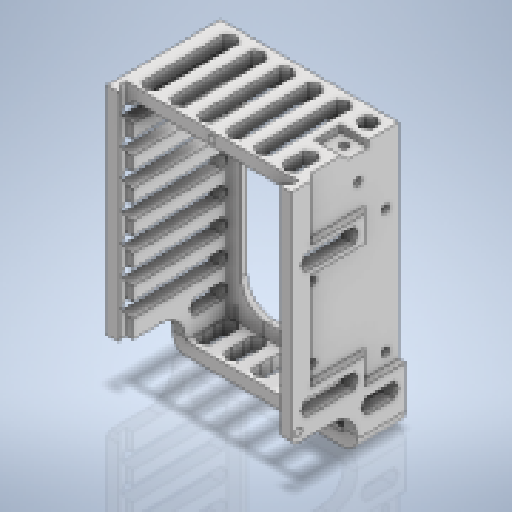
# Autodesk Inventor part: corpo
Saved by Autodesk Inventor 2024.3 (Build 283343000, 343)
## iProperties
Created: 2024-03-03
Part Number: corpo
Material: Genérico
Document SubType Name: Modeling
Designer: joaov
Density: 1 g/cm^3
Appearance: Padrão
Author: joaov
Autodesk Inventor part; units mm, degrees
note: some values were not read from the file. Chosen so that the rebuilt part matches the saved one: edges of "Chanfro6".
(part 1 of 2)
ref_plane "YZ Plane" through (0, 0, 0) normal (1, 0, 0) x (0, 1, 0)
ref_plane "XZ Plane" through (0, 0, 0) normal (0, 1, 0) x (-1, 0, 0)
ref_plane "XY Plane" through (0, 0, 0) normal (0, 0, 1) x (1, 0, 0)
sketch "Esboço1" plane through (0, 0, 0) normal (0, 0, 1) x (1, 0, 0)
  line L0 (0, 0) -> (59, 0)
  line L1 (59, 0) -> (59, 87)
  line L2 (59, 87) -> (0, 87)
  line L3 (0, 87) -> (0, 0)
  line L4 (59, 43.5) -> (63.8, 43.5)
  line L5 (29.5, 87) -> (29.5, 91.8)
  line L6 (-4.8, -4.8) -> (63.8, -4.8)
  line L7 (63.8, -4.8) -> (63.8, 91.8)
  line L8 (63.8, 91.8) -> (-4.8, 91.8)
  line L9 (-4.8, 91.8) -> (-4.8, -4.8)
  line L10 (-4.8, -4.8) -> (63.8, 91.8) construction
  line L11 (63.8, -4.8) -> (-4.8, 91.8) construction
  point P0 (29.5, 43.5)
  dimension "d0" = 59
  dimension "d1" = 87
  dimension "d2" = 4.8
  dimension "d3" = 4.8
  constraints: 24 end point, 4 midpoint, 4 perpendicular, 3 horizontal, 2 parallel, 1 vertical
  measures "d0" distance of L0.start L0.end
  measures "d1" distance of L0.end L1.end
  measures "d2" distance of L4.start L4.end
  measures "d3" distance of L5.start L5.end
extrude "paredes" add sketch "Esboço1" along normal blind 35 contours L0 L1 L4 L7 L6 L9 L8 L5 L2 L3 | L1 L2 L5 L8 L7 L4
sketch "Esboço2" plane through (0, 0, 0) normal (0, 0, -1) x (-1, 0, 0)
  line L0 (4.8, 91.8) -> (4.8, -4.8) projected
  line L1 (-63.8, 91.8) -> (4.8, 91.8)
  line L2 (4.8, 91.8) -> (4.8, -4.8)
  line L3 (4.8, -4.8) -> (-63.8, -4.8)
  line L4 (-63.8, -4.8) -> (-63.8, 91.8)
  point P0 (0, 0)
  constraints: 8 end point, 2 parallel, 1 horizontal, 1 perpendicular
extrude "base" add sketch "Esboço2" along normal blind 2.4
sketch "Esboço3" plane through (-4.8, -4.8, 35) normal (0, -1, 0) x (1, 0, 0)
  line L0 (0, -37.4) -> (0, 0) projected
  line L1 (0, 0) -> (2.4, 0)
  line L2 (68.6, 0) -> (0, 0) projected
  line L3 (0, 0) -> (0, 4.8)
  line L4 (0, 4.8) -> (4.3, 4.8)
  line L5 (2.4, 2.4) -> (4.3, 4.3)
  line L6 (2.4, 0) -> (2.4, 2.4)
  line L7 (4.3, 4.8) -> (4.3, 4.3)
  line L8 (34.3, 0) -> (34.3, 4.8)
  line L9 (68.6, 0) -> (66.2, 0)
  line L10 (68.6, 0) -> (68.6, 4.8)
  line L11 (68.6, 4.8) -> (64.3, 4.8)
  line L12 (66.2, 2.4) -> (64.3, 4.3)
  line L13 (66.2, 0) -> (66.2, 2.4)
  line L14 (64.3, 4.8) -> (64.3, 4.3)
  point P0 (4.8, -35)
  dimension "d27" = 0.5
  constraints: 26 end point, 5 symmetric about line, 2 vertical, 1 midpoint, 1 perpendicular, 1 point on line
  measures "d27" distance of L12.end L11.end
extrude "Extrusão3" add sketch "Esboço3" against normal blind 96.6
sketch "Esboço4" plane through (0, 0, 35) normal (0, 0, 1) x (1, 0, 0)
  line L0 (59, 87) -> (0, 87)
  line L1 (29.5, 87) -> (29.5, 91.8)
  line L2 (63.8, 91.8) -> (-4.8, 91.8)
  line L3 (29.5, 89.4) -> (51, 89.4)
  line L4 (29.5, 87) -> (29.5, 91.8)
  line L5 (29.5, 89.4) -> (8, 89.4)
  line L6 (29.5, 89.4) -> (51, 89.4)
  circle A0 centre (51, 89.4) radius 1.45
  circle A1 centre (8, 89.4) radius 1.45
  line L7 (59.5, -4.8) -> (59.5, 91.8) projected
  line L8 (-0.5, -4.8) -> (-0.5, 91.8) projected
  circle A2 centre (29.5, 89.4) radius 1.45
  point P0 (0, 0)
  point P1 (59, 0)
  point P2 (63.8, -4.8)
  point P3 (-4.8, -4.8)
  dimension "d161" = 8.5
  dimension "d162" = 8.5
  dimension "d255" = 2.9
  dimension "d265" = 2.9
  dimension "d266" = 2.9
  constraints: 14 end point, 3 centre point, 3 coincident
  measures "d161" distance from line of L3.end L7
  measures "d162" distance from line of L5.end L8
  measures "d255" diameter of A2
  measures "d265" diameter of A1
  measures "d266" diameter of A0
extrude "Extrusão4" cut sketch "Esboço4" against normal blind 10 contours A2 L5 L1 | L1 L3 A2 | L5 A2 L1 | L1 A2 L3
sketch "Esboço5" plane through (-4.8, -4.8, -2.4) normal (0, -1, 0) x (1, 0, 0)
  line L0 (0, 0) -> (68.6, 0) projected
  line L1 (20.3, 17.9) -> (10.3, 17.9)
  line L2 (20.3, 17.9) -> (30.3, 17.9)
  line L3 (30.3, 17.9) -> (20.3, 27.9)
  line L4 (20.3, 27.9) -> (10.3, 17.9)
  line L5 (66.2, 37.4) -> (2.4, 37.4) projected
  line L6 (2.4, 37.4) -> (2.4, 17.9)
  line L7 (4.8, 2.4) -> (4.8, 37.4) projected
  line L8 (2.4, 17.9) -> (66.2, 17.9)
  line L9 (66.2, 17.9) -> (66.2, 37.4)
  line L10 (66.2, 37.4) -> (2.4, 37.4)
  line L11 (0, 42.2) -> (4.3, 42.2) projected
  line L12 (68.6, 0) -> (68.6, 42.2) projected
  line L13 (0, 42.2) -> (68.6, 42.2)
  line L14 (68.6, 42.2) -> (68.6, 17.9)
  line L15 (68.6, 17.9) -> (0, 17.9)
  line L16 (0, 17.9) -> (0, 42.2)
  point P0 (2.4, 17.9)
  dimension "d36" = 10
  dimension "d37" = 10
  dimension "d38" = 45
  constraints: 24 end point, 5 perpendicular, 3 horizontal, 3 parallel, 1 point on line
  measures "d36" distance of L1.start L1.end
  measures "d37" distance of L1.start L2.end
  measures "d38" angle of L3 L2
extrude "Extrusão5" cut sketch "Esboço5" against normal blind 14.8
sketch "Esboço10" plane through (63.8, -4.8, -2.4) normal (1, 0, 0) x (0, 0, -1)
  line L0 (-7.5, 75.981) -> (0, 75.981)
  line L1 (-7.5, 20.619) -> (0, 20.619)
  line L2 (-7.5, 75.981) -> (-15.2, 75.981)
  line L3 (-15.2, 75.981) -> (-15.2, 66.3)
  line L4 (-15.2, 30.3) -> (-15.2, 20.619)
  line L5 (-15.2, 20.619) -> (-7.5, 20.619)
  line L6 (0, 75.981) -> (0, 20.619)
  line L7 (-18.58, 30.3) -> (-15.2, 30.3)
  line L8 (-18.58, 66.3) -> (-15.2, 66.3)
  line L9 (-35.3, 30.3) -> (-35.3, 66.3)
  line L10 (-18.58, 66.3) -> (-35.3, 66.3)
  line L11 (-18.58, 30.3) -> (-35.3, 30.3)
  line L12 (0, 0) -> (0, 96.6) projected
  line L13 (0, 96.6) -> (0, 0)
  point P0 (-2.4, 4.8)
  point P1 (-35.0419, -145.2014)
  constraints: 26 end point, 6 perpendicular, 1 collinear
extrude "Extrusão9" cut sketch "Esboço10" against normal blind 2.5
sketch "Esboço11" plane through (61.3, -4.8, -2.4) normal (1, 0, 0) x (0, 0, -1)
  line L0 (-15.2, 66.3) -> (-15.2, 75.981)
  line L1 (-15.2, 71.1405) -> (-15, 71.1405)
  line L2 (-15.2, 71.1405) -> (-15.2, 70.9405) construction
  line L3 (-15.2, 75.981) -> (0, 75.981)
  line L4 (-7.6, 75.981) -> (-7.6, 75.781)
  line L5 (-7.6, 75.981) -> (-7.6, 75.781) construction
  line L6 (0, 75.981) -> (0, 20.619)
  line L7 (0, 75.781) -> (-10, 75.781)
  line L8 (-5, 75.781) -> (-5, 72.781)
  line L9 (-5, 72.781) -> (-5, 71.281)
  line L10 (0, 48.3) -> (-3.0797, 48.3)
  line L11 (-15.2, 75.981) -> (0, 75.981)
  line L12 (-35.3, 66.3) -> (-15.2, 66.3)
  line L13 (-35.3, 30.3) -> (-35.3, 66.3)
  line L14 (-35.3, 66.3) -> (-35.3, 30.3)
  line L15 (-35.3, 48.3) -> (-32.1, 48.3)
  line L16 (-32.1, 66.3) -> (-32.1, 63.1)
  line L17 (-32.1, 63.1) -> (-32.1, 61.6)
  line L18 (0, 48.3) -> (-35.3, 48.3)
  line L19 (-17.65, 48.3) -> (-17.65, 54.676)
  line L20 (-35.3, 30.3) -> (-35.3, 66.3) projected
  line L21 (-35.3, 48.3) -> (-37.5242, 48.3)
  line L22 (-5, 25.319) -> (-15.2, 25.319)
  line L23 (-15.2, 20.619) -> (-15.2, 30.3) projected
  circle A0 centre (-5, 25.319) radius 1.45
  circle A1 centre (-32.1, 35) radius 1.45
  circle A2 centre (-32.1, 61.6) radius 1.45
  circle A3 centre (-5, 71.281) radius 1.45
  point P0 (-2.4, 4.8)
  point P1 (33.1289, 48.912)
  dimension "d58" = 90
  dimension "d59" = 0.2
  dimension "d61" = 3
  dimension "d62" = 1.5
  dimension "d64" = 3.2
  dimension "d65" = 3.2
  dimension "d66" = 1.5
  dimension "d260" = 2.9
  dimension "d261" = 2.9
  dimension "d262" = 2.9
  dimension "d263" = 2.9
  constraints: 44 end point, 8 midpoint, 4 centre point, 4 point on line, 2 equal length, 2 horizontal, 1 coincident, 1 perpendicular
  measures "d58" angle of L2 L1
  measures "d59" distance of L1.start L1.end
  measures "d61" distance of L8.start L8.end
  measures "d62" distance of L8.end L9.end
  measures "d64" distance of L15.start L15.end
  measures "d65" distance of L16.start L16.end
  measures "d66" distance of L16.end L17.end
  measures "d260" diameter of A0
  measures "d261" diameter of A1
  measures "d262" diameter of A2
  measures "d263" diameter of A3
extrude "Extrusão10" cut sketch "Esboço11" against normal blind 8.25 contours A0 | A1 | A2 | A3
chamfer "Chanfro1" distance 2.5 angle 45 1 edges at (61.3, 43.5, 32.9)
chamfer "Chanfro2" distance 2.5 angle 45 2 edges at (61.3, 20.6595, 12.8) (61.3, 66.3405, 12.8)
sketch "Esboço14" plane through (63.8, 91.8, 39.8) normal (1, 0, 0) x (0, 0, -1)
  line L0 (0, 0) -> (42.2, 0) projected
  line L1 (10.6384, 0) -> (38.6384, 0) construction
  line L2 (2.4, -81.8) -> (2.4, 0) projected
  line L3 (2.4, 0) -> (2.4, -30.2771)
  line L4 (2.4, -30.2771) -> (4.8, -30.2771)
  line L5 (4.8, -4.8) -> (4.8, -81.8) projected
  line L6 (4.8, -30.2771) -> (4.8, 0)
  line L7 (6.9, -66.3) -> (6.9, -30.3) projected
  line L8 (6.9, -20.619) -> (6.9, 0)
  line L9 (27, -30.3) -> (27, -20.619) projected
  line L10 (27, -20.619) -> (6.9, -20.619)
  line L11 (42.2, 0) -> (42.2, -20.619) projected
  line L12 (42.2, -20.619) -> (27, -20.619)
  line L13 (42.2, -20.619) -> (42.2, 0)
  line L14 (0, 0) -> (6.9, 0)
  line L15 (42.2, 0) -> (0, 0) projected
  line L16 (6.9, 0) -> (42.2, 0)
  point P0 (39.8, -91.8)
  dimension "d101" = 35.3
  dimension "d102" = 20.619
  constraints: 20 end point, 4 perpendicular, 4 point on line, 3 horizontal, 2 collinear, 1 vertical
  measures "d101" distance of L0.end L8.end
  measures "d102" distance of L0.end L11.end
extrude "Extrusão11" cut sketch "Esboço14" against normal blind 2.5 contours L0 L11 L12 L10 L8
chamfer "Chanfro3" distance 2.5 angle 45 1 edges at (61.3, 81.4905, 32.9)
sketch "Esboço17" plane through (-2.4, 91.8, 35) normal (0, 1, 0) x (1, 0, 0)
  line L0 (53.7, 21) -> (53.7, 16)
  line L1 (53.7, 16) -> (63.7, 16)
  line L2 (63.7, 16) -> (63.7, 26)
  line L3 (63.7, 26) -> (53.7, 26)
  line L4 (53.7, 26) -> (53.7, 21)
  point P0 (63.7, 4.6)
  constraints: 10 end point, 1 horizontal, 1 perpendicular, 1 vertical
extrude "Extrusão14" cut sketch "Esboço17" against normal blind 2.5
chamfer "Chanfro6" distance 2.5 angle 45 1 edges at (56.3, 89.3, 19)
sketch "Esboço18" plane through (-2.4, 89.3, 35) normal (0, 1, 0) x (1, 0, 0)
  line L0 (2.4, 0) -> (61.4, 0) projected
  line L1 (-2.4, 37.4) -> (63.7, 37.4) projected
  circle A0 centre (58.7, 22.25) radius 1.45
  point P0 (10.1, 26)
  point P1 (0.1, 18.5)
  dimension "d264" = 2.9
  constraints: 1 centre point
  measures "d264" diameter of A0
extrude "Extrusão15" cut sketch "Esboço18" against normal blind 2.5
fillet "Arredondamento2" radius 9 2 edges at (-2.4, 10, 15.5) (61.4, 10, 15.5)
fillet "Arredondamento3" radius 5 2 edges at (-4.8, -4.8, 6.55) (63.8, -4.8, 6.55)
sketch "Esboço24" plane through (-4.8, 91.8, -2.4) normal (-1, 0, 0) x (0, 0, 1)
  line L0 (28.975, -77) -> (35, -77)
  line L1 (-2.4, -30.2362) -> (2.4, -30.2362) construction
  line L2 (2.4, -9.5605) -> (4.03, -6.7373)
  line L3 (4.03, -6.7373) -> (7.29, -6.7373)
  line L4 (7.29, -6.7373) -> (8.92, -9.5605)
  line L5 (8.92, -9.5605) -> (7.29, -12.3838)
  line L6 (7.29, -12.3838) -> (4.03, -12.3838)
  line L7 (4.03, -12.3838) -> (2.4, -9.5605)
  line L8 (2.4, -20.007) -> (4.03, -17.1838)
  line L9 (4.03, -17.1838) -> (7.29, -17.1838)
  line L10 (7.29, -17.1838) -> (8.92, -20.007)
  line L11 (8.92, -20.007) -> (7.29, -22.8303)
  line L12 (7.29, -22.8303) -> (4.03, -22.8303)
  line L13 (4.03, -22.8303) -> (2.4, -20.007)
  line L14 (2.4, -30.4535) -> (4.03, -27.6303)
  line L15 (4.03, -27.6303) -> (7.29, -27.6303)
  line L16 (7.29, -27.6303) -> (8.92, -30.4535)
  line L17 (8.92, -30.4535) -> (7.29, -33.2768)
  line L18 (7.29, -33.2768) -> (4.03, -33.2768)
  line L19 (4.03, -33.2768) -> (2.4, -30.4535)
  line L20 (7.29, -43.7232) -> (4.03, -43.7232)
  line L21 (8.92, -40.9) -> (7.29, -43.7232)
  line L22 (4.03, -43.7232) -> (2.4, -40.9)
  line L23 (2.4, -40.9) -> (4.03, -38.0768)
  line L24 (4.03, -38.0768) -> (7.29, -38.0768)
  line L25 (7.29, -38.0768) -> (8.92, -40.9)
  line L26 (2.4, -51.3465) -> (4.03, -48.5232)
  line L27 (4.03, -48.5232) -> (7.29, -48.5232)
  line L28 (7.29, -48.5232) -> (8.92, -51.3465)
  line L29 (8.92, -51.3465) -> (7.29, -54.1697)
  line L30 (7.29, -54.1697) -> (4.03, -54.1697)
  line L31 (4.03, -54.1697) -> (2.4, -51.3465)
  line L32 (7.29, -64.6162) -> (4.03, -64.6162)
  line L33 (8.92, -61.793) -> (7.29, -64.6162)
  line L34 (4.03, -64.6162) -> (2.4, -61.793)
  line L35 (2.4, -61.793) -> (4.03, -58.9697)
  line L36 (4.03, -58.9697) -> (7.29, -58.9697)
  line L37 (7.29, -58.9697) -> (8.92, -61.793)
  line L38 (4.03, -69.4162) -> (7.29, -69.4162)
  line L39 (2.4, -72.2395) -> (4.03, -69.4162)
  line L40 (4.03, -75.0627) -> (2.4, -72.2395)
  line L41 (7.29, -69.4162) -> (8.92, -72.2395)
  line L42 (7.29, -75.0627) -> (4.03, -75.0627)
  line L43 (8.92, -72.2395) -> (7.29, -75.0627)
  line L44 (4.03, -79.8627) -> (7.29, -79.8627)
  line L45 (4.03, -85.5092) -> (2.4, -82.6859)
  line L46 (7.29, -85.5092) -> (4.03, -85.5092)
  line L47 (2.4, -82.6859) -> (4.03, -79.8627)
  line L48 (7.29, -79.8627) -> (8.92, -82.6859)
  line L49 (8.92, -82.6859) -> (7.29, -85.5092)
  line L50 (8.92, -9.5605) -> (9.92, -9.5605)
  line L51 (9.92, -9.5605) -> (11.55, -6.7373)
  line L52 (11.55, -6.7373) -> (14.81, -6.7373)
  line L53 (14.81, -6.7373) -> (16.44, -9.5605)
  line L54 (16.44, -9.5605) -> (14.81, -12.3838)
  line L55 (14.81, -12.3838) -> (11.55, -12.3838)
  line L56 (11.55, -12.3838) -> (9.92, -9.5605)
  line L57 (14.81, -22.8303) -> (11.55, -22.8303)
  line L58 (16.44, -20.007) -> (14.81, -22.8303)
  line L59 (11.55, -22.8303) -> (9.92, -20.007)
  line L60 (9.92, -20.007) -> (11.55, -17.1838)
  line L61 (11.55, -17.1838) -> (14.81, -17.1838)
  line L62 (14.81, -17.1838) -> (16.44, -20.007)
  line L63 (9.92, -30.4535) -> (11.55, -27.6303)
  line L64 (11.55, -27.6303) -> (14.81, -27.6303)
  line L65 (14.81, -27.6303) -> (16.44, -30.4535)
  line L66 (16.44, -30.4535) -> (14.81, -33.2768)
  line L67 (14.81, -33.2768) -> (11.55, -33.2768)
  line L68 (11.55, -33.2768) -> (9.92, -30.4535)
  line L69 (14.81, -43.7232) -> (11.55, -43.7232)
  line L70 (16.44, -40.9) -> (14.81, -43.7232)
  line L71 (11.55, -43.7232) -> (9.92, -40.9)
  line L72 (14.81, -38.0768) -> (16.44, -40.9)
  line L73 (11.55, -38.0768) -> (14.81, -38.0768)
  line L74 (9.92, -40.9) -> (11.55, -38.0768)
  line L75 (9.92, -51.3465) -> (11.55, -48.5232)
  line L76 (11.55, -48.5232) -> (14.81, -48.5232)
  line L77 (14.81, -48.5232) -> (16.44, -51.3465)
  line L78 (16.44, -51.3465) -> (14.81, -54.1697)
  line L79 (14.81, -54.1697) -> (11.55, -54.1697)
  line L80 (11.55, -54.1697) -> (9.92, -51.3465)
  line L81 (14.81, -64.6162) -> (11.55, -64.6162)
  line L82 (16.44, -61.793) -> (14.81, -64.6162)
  line L83 (11.55, -64.6162) -> (9.92, -61.793)
  line L84 (14.81, -58.9697) -> (16.44, -61.793)
  line L85 (11.55, -58.9697) -> (14.81, -58.9697)
  line L86 (9.92, -61.793) -> (11.55, -58.9697)
  line L87 (11.55, -69.4162) -> (14.81, -69.4162)
  line L88 (11.55, -75.0627) -> (9.92, -72.2395)
  line L89 (14.81, -75.0627) -> (11.55, -75.0627)
  line L90 (9.92, -72.2395) -> (11.55, -69.4162)
  line L91 (14.81, -69.4162) -> (16.44, -72.2395)
  line L92 (16.44, -72.2395) -> (14.81, -75.0627)
  line L93 (11.55, -79.8627) -> (14.81, -79.8627)
  line L94 (14.81, -79.8627) -> (16.44, -82.6859)
  line L95 (9.92, -82.6859) -> (11.55, -79.8627)
  line L96 (16.44, -82.6859) -> (14.81, -85.5092)
  line L97 (14.81, -85.5092) -> (11.55, -85.5092)
  line L98 (11.55, -85.5092) -> (9.92, -82.6859)
  line L99 (16.44, -9.5605) -> (17.44, -9.5605)
  line L100 (17.44, -9.5605) -> (19.07, -6.7373)
  line L101 (19.07, -6.7373) -> (22.33, -6.7373)
  line L102 (22.33, -6.7373) -> (23.96, -9.5605)
  line L103 (23.96, -9.5605) -> (22.33, -12.3838)
  line L104 (22.33, -12.3838) -> (19.07, -12.3838)
  line L105 (19.07, -12.3838) -> (17.44, -9.5605)
  line L106 (22.33, -22.8303) -> (19.07, -22.8303)
  line L107 (23.96, -20.007) -> (22.33, -22.8303)
  line L108 (19.07, -22.8303) -> (17.44, -20.007)
  line L109 (17.44, -20.007) -> (19.07, -17.1838)
  line L110 (19.07, -17.1838) -> (22.33, -17.1838)
  line L111 (22.33, -17.1838) -> (23.96, -20.007)
  line L112 (17.44, -30.4535) -> (19.07, -27.6303)
  line L113 (19.07, -27.6303) -> (22.33, -27.6303)
  line L114 (22.33, -27.6303) -> (23.96, -30.4535)
  line L115 (23.96, -30.4535) -> (22.33, -33.2768)
  line L116 (22.33, -33.2768) -> (19.07, -33.2768)
  line L117 (19.07, -33.2768) -> (17.44, -30.4535)
  line L118 (22.33, -43.7232) -> (19.07, -43.7232)
  line L119 (23.96, -40.9) -> (22.33, -43.7232)
  line L120 (19.07, -43.7232) -> (17.44, -40.9)
  line L121 (22.33, -38.0768) -> (23.96, -40.9)
  line L122 (19.07, -38.0768) -> (22.33, -38.0768)
  line L123 (17.44, -40.9) -> (19.07, -38.0768)
  line L124 (17.44, -51.3465) -> (19.07, -48.5232)
  line L125 (19.07, -48.5232) -> (22.33, -48.5232)
  line L126 (22.33, -48.5232) -> (23.96, -51.3465)
  line L127 (23.96, -51.3465) -> (22.33, -54.1697)
  line L128 (22.33, -54.1697) -> (19.07, -54.1697)
  line L129 (19.07, -54.1697) -> (17.44, -51.3465)
  line L130 (22.33, -64.6162) -> (19.07, -64.6162)
  line L131 (23.96, -61.793) -> (22.33, -64.6162)
  line L132 (19.07, -64.6162) -> (17.44, -61.793)
  line L133 (22.33, -58.9697) -> (23.96, -61.793)
  line L134 (19.07, -58.9697) -> (22.33, -58.9697)
  line L135 (17.44, -61.793) -> (19.07, -58.9697)
  line L136 (19.07, -69.4162) -> (22.33, -69.4162)
  line L137 (19.07, -75.0627) -> (17.44, -72.2395)
  line L138 (22.33, -75.0627) -> (19.07, -75.0627)
  line L139 (17.44, -72.2395) -> (19.07, -69.4162)
  line L140 (22.33, -69.4162) -> (23.96, -72.2395)
  line L141 (23.96, -72.2395) -> (22.33, -75.0627)
  line L142 (23.96, -9.5605) -> (24.96, -9.5605)
  line L143 (24.96, -9.5605) -> (26.59, -6.7373)
  line L144 (26.59, -6.7373) -> (29.85, -6.7373)
  line L145 (29.85, -6.7373) -> (31.48, -9.5605)
  line L146 (31.48, -9.5605) -> (29.85, -12.3838)
  line L147 (29.85, -12.3838) -> (26.59, -12.3838)
  line L148 (26.59, -12.3838) -> (24.96, -9.5605)
  line L149 (29.85, -22.8303) -> (26.59, -22.8303)
  line L150 (31.48, -20.007) -> (29.85, -22.8303)
  line L151 (26.59, -22.8303) -> (24.96, -20.007)
  line L152 (24.96, -20.007) -> (26.59, -17.1838)
  line L153 (26.59, -17.1838) -> (29.85, -17.1838)
  line L154 (29.85, -17.1838) -> (31.48, -20.007)
  line L155 (24.96, -30.4535) -> (26.59, -27.6303)
  line L156 (26.59, -27.6303) -> (29.85, -27.6303)
  line L157 (29.85, -27.6303) -> (31.48, -30.4535)
  line L158 (31.48, -30.4535) -> (29.85, -33.2768)
  line L159 (29.85, -33.2768) -> (26.59, -33.2768)
  line L160 (26.59, -33.2768) -> (24.96, -30.4535)
  line L161 (29.85, -43.7232) -> (26.59, -43.7232)
  line L162 (31.48, -40.9) -> (29.85, -43.7232)
  line L163 (26.59, -43.7232) -> (24.96, -40.9)
  line L164 (29.85, -38.0768) -> (31.48, -40.9)
  line L165 (26.59, -38.0768) -> (29.85, -38.0768)
  line L166 (24.96, -40.9) -> (26.59, -38.0768)
  line L167 (24.96, -51.3465) -> (26.59, -48.5232)
  line L168 (26.59, -48.5232) -> (29.85, -48.5232)
  line L169 (29.85, -48.5232) -> (31.48, -51.3465)
  line L170 (31.48, -51.3465) -> (29.85, -54.1697)
  line L171 (29.85, -54.1697) -> (26.59, -54.1697)
  line L172 (26.59, -54.1697) -> (24.96, -51.3465)
  line L173 (29.85, -64.6162) -> (26.59, -64.6162)
  line L174 (31.48, -61.793) -> (29.85, -64.6162)
  line L175 (26.59, -64.6162) -> (24.96, -61.793)
  line L176 (29.85, -58.9697) -> (31.48, -61.793)
  line L177 (26.59, -58.9697) -> (29.85, -58.9697)
  line L178 (24.96, -61.793) -> (26.59, -58.9697)
  line L179 (26.59, -69.4162) -> (29.85, -69.4162)
  line L180 (26.59, -75.0627) -> (24.96, -72.2395)
  line L181 (29.85, -75.0627) -> (26.59, -75.0627)
  line L182 (24.96, -72.2395) -> (26.59, -69.4162)
  line L183 (29.85, -69.4162) -> (31.48, -72.2395)
  line L184 (31.48, -72.2395) -> (29.85, -75.0627)
  line L185 (31.48, -9.5605) -> (32.48, -9.5605)
  line L186 (2.4, -9.5605) -> (0, -9.5605)
  line L187 (37.37, -33.2768) -> (34.11, -33.2768)
  line L188 (34.11, -33.2768) -> (32.48, -30.4535)
  line L189 (34.11, -27.6303) -> (37.37, -27.6303)
  line L190 (32.48, -30.4535) -> (34.11, -27.6303)
  line L191 (34.11, -38.0768) -> (37.37, -38.0768)
  line L192 (37.37, -38.0768) -> (39, -40.9)
  line L193 (32.48, -40.9) -> (34.11, -38.0768)
  line L194 (39, -40.9) -> (37.37, -43.7232)
  line L195 (37.37, -43.7232) -> (34.11, -43.7232)
  line L196 (34.11, -43.7232) -> (32.48, -40.9)
  line L197 (37.37, -27.6303) -> (39, -30.4535)
  line L198 (39, -30.4535) -> (37.37, -33.2768)
  line L199 (34.11, -48.5232) -> (37.37, -48.5232)
  line L200 (32.48, -51.3465) -> (34.11, -48.5232)
  line L201 (39, -51.3465) -> (37.37, -54.1697)
  line L202 (37.37, -54.1697) -> (34.11, -54.1697)
  line L203 (34.11, -54.1697) -> (32.48, -51.3465)
  line L204 (34.11, -58.9697) -> (37.37, -58.9697)
  line L205 (32.48, -61.793) -> (34.11, -58.9697)
  line L206 (37.37, -58.9697) -> (39, -61.793)
  line L207 (34.11, -64.6162) -> (32.48, -61.793)
  line L208 (37.37, -64.6162) -> (34.11, -64.6162)
  line L209 (39, -61.793) -> (37.37, -64.6162)
  line L210 (37.37, -48.5232) -> (39, -51.3465)
  line L211 (34.11, -69.4162) -> (37.37, -69.4162)
  line L212 (32.48, -72.2395) -> (34.11, -69.4162)
  line L213 (37.37, -69.4162) -> (39, -72.2395)
  line L214 (37.37, -75.0627) -> (34.11, -75.0627)
  line L215 (39, -72.2395) -> (37.37, -75.0627)
  line L216 (34.11, -75.0627) -> (32.48, -72.2395)
  line L217 (32.48, -9.5605) -> (34.11, -6.7373)
  line L218 (34.11, -6.7373) -> (37.37, -6.7373)
  line L219 (37.37, -6.7373) -> (39, -9.5605)
  line L220 (39, -9.5605) -> (37.37, -12.3838)
  line L221 (37.37, -12.3838) -> (34.11, -12.3838)
  line L222 (34.11, -12.3838) -> (32.48, -9.5605)
  line L223 (37.37, -22.8303) -> (34.11, -22.8303)
  line L224 (39, -20.007) -> (37.37, -22.8303)
  line L225 (34.11, -22.8303) -> (32.48, -20.007)
  line L226 (32.48, -20.007) -> (34.11, -17.1838)
  line L227 (34.11, -17.1838) -> (37.37, -17.1838)
  line L228 (37.37, -17.1838) -> (39, -20.007)
  line L229 (39, -9.5605) -> (40, -9.5605)
  line L230 (4.03, -6.7373) -> (37.37, -6.7373)
  line L231 (4.03, -12.3838) -> (37.37, -12.3838)
  line L232 (2.4, -20.007) -> (4.03, -17.1838)
  line L233 (4.03, -17.1838) -> (7.29, -17.1838)
  line L234 (7.29, -17.1838) -> (8.92, -20.007)
  line L235 (8.92, -20.007) -> (7.29, -22.8303)
  line L236 (7.29, -22.8303) -> (4.03, -22.8303)
  line L237 (4.03, -22.8303) -> (2.4, -20.007)
  line L238 (8.92, -20.007) -> (9.92, -20.007)
  line L239 (9.92, -20.007) -> (11.55, -17.1838)
  line L240 (11.55, -17.1838) -> (14.81, -17.1838)
  line L241 (14.81, -17.1838) -> (16.44, -20.007)
  line L242 (16.44, -20.007) -> (14.81, -22.8303)
  line L243 (14.81, -22.8303) -> (11.55, -22.8303)
  line L244 (11.55, -22.8303) -> (9.92, -20.007)
  line L245 (16.44, -20.007) -> (17.44, -20.007)
  line L246 (17.44, -20.007) -> (19.07, -17.1838)
  line L247 (19.07, -17.1838) -> (22.33, -17.1838)
  line L248 (22.33, -17.1838) -> (23.96, -20.007)
  line L249 (23.96, -20.007) -> (22.33, -22.8303)
  line L250 (22.33, -22.8303) -> (19.07, -22.8303)
  line L251 (19.07, -22.8303) -> (17.44, -20.007)
  line L252 (23.96, -20.007) -> (24.96, -20.007)
  line L253 (24.96, -20.007) -> (26.59, -17.1838)
  line L254 (26.59, -17.1838) -> (29.85, -17.1838)
  line L255 (29.85, -17.1838) -> (31.48, -20.007)
  line L256 (31.48, -20.007) -> (29.85, -22.8303)
  line L257 (29.85, -22.8303) -> (26.59, -22.8303)
  line L258 (26.59, -22.8303) -> (24.96, -20.007)
  line L259 (31.48, -20.007) -> (32.48, -20.007)
  line L260 (2.4, -20.007) -> (0, -20.007)
  line L261 (34.11, -22.8303) -> (32.48, -20.007)
  line L262 (32.48, -20.007) -> (34.11, -17.1838)
  line L263 (37.37, -22.8303) -> (34.11, -22.8303)
  line L264 (34.11, -17.1838) -> (37.37, -17.1838)
  line L265 (37.37, -17.1838) -> (39, -20.007)
  line L266 (39, -20.007) -> (37.37, -22.8303)
  line L267 (39, -20.007) -> (40, -20.007)
  line L268 (4.03, -17.1838) -> (37.37, -17.1838)
  line L269 (4.03, -22.8303) -> (37.37, -22.8303)
  line L270 (2.4, -30.4535) -> (4.03, -27.6303)
  line L271 (4.03, -27.6303) -> (7.29, -27.6303)
  line L272 (7.29, -27.6303) -> (8.92, -30.4535)
  line L273 (8.92, -30.4535) -> (7.29, -33.2768)
  line L274 (7.29, -33.2768) -> (4.03, -33.2768)
  line L275 (4.03, -33.2768) -> (2.4, -30.4535)
  line L276 (8.92, -30.4535) -> (9.92, -30.4535)
  line L277 (9.92, -30.4535) -> (11.55, -27.6303)
  line L278 (11.55, -27.6303) -> (14.81, -27.6303)
  line L279 (14.81, -27.6303) -> (16.44, -30.4535)
  line L280 (16.44, -30.4535) -> (14.81, -33.2768)
  line L281 (14.81, -33.2768) -> (11.55, -33.2768)
  line L282 (11.55, -33.2768) -> (9.92, -30.4535)
  line L283 (16.44, -30.4535) -> (17.44, -30.4535)
  line L284 (17.44, -30.4535) -> (19.07, -27.6303)
  line L285 (19.07, -27.6303) -> (22.33, -27.6303)
  line L286 (22.33, -27.6303) -> (23.96, -30.4535)
  line L287 (23.96, -30.4535) -> (22.33, -33.2768)
  line L288 (22.33, -33.2768) -> (19.07, -33.2768)
  line L289 (19.07, -33.2768) -> (17.44, -30.4535)
  line L290 (23.96, -30.4535) -> (24.96, -30.4535)
  line L291 (24.96, -30.4535) -> (26.59, -27.6303)
  line L292 (26.59, -27.6303) -> (29.85, -27.6303)
  line L293 (29.85, -27.6303) -> (31.48, -30.4535)
  line L294 (31.48, -30.4535) -> (29.85, -33.2768)
  line L295 (29.85, -33.2768) -> (26.59, -33.2768)
  line L296 (26.59, -33.2768) -> (24.96, -30.4535)
  line L297 (31.48, -30.4535) -> (32.48, -30.4535)
  line L298 (2.4, -30.4535) -> (0, -30.4535)
  line L299 (34.11, -33.2768) -> (32.48, -30.4535)
  line L300 (32.48, -30.4535) -> (34.11, -27.6303)
  line L301 (37.37, -33.2768) -> (34.11, -33.2768)
  line L302 (34.11, -27.6303) -> (37.37, -27.6303)
  line L303 (37.37, -27.6303) -> (39, -30.4535)
  line L304 (39, -30.4535) -> (37.37, -33.2768)
  line L305 (39, -30.4535) -> (40, -30.4535)
  line L306 (4.03, -27.6303) -> (37.37, -27.6303)
  line L307 (4.03, -33.2768) -> (37.37, -33.2768)
  line L308 (2.4, -40.9) -> (4.03, -38.0768)
  line L309 (4.03, -38.0768) -> (7.29, -38.0768)
  line L310 (7.29, -38.0768) -> (8.92, -40.9)
  line L311 (8.92, -40.9) -> (7.29, -43.7232)
  line L312 (7.29, -43.7232) -> (4.03, -43.7232)
  line L313 (4.03, -43.7232) -> (2.4, -40.9)
  line L314 (8.92, -40.9) -> (9.92, -40.9)
  line L315 (9.92, -40.9) -> (11.55, -38.0768)
  line L316 (11.55, -38.0768) -> (14.81, -38.0768)
  line L317 (14.81, -38.0768) -> (16.44, -40.9)
  line L318 (16.44, -40.9) -> (14.81, -43.7232)
  line L319 (14.81, -43.7232) -> (11.55, -43.7232)
  line L320 (11.55, -43.7232) -> (9.92, -40.9)
  line L321 (16.44, -40.9) -> (17.44, -40.9)
  line L322 (17.44, -40.9) -> (19.07, -38.0768)
  line L323 (19.07, -38.0768) -> (22.33, -38.0768)
  line L324 (22.33, -38.0768) -> (23.96, -40.9)
  line L325 (23.96, -40.9) -> (22.33, -43.7232)
  line L326 (22.33, -43.7232) -> (19.07, -43.7232)
  line L327 (19.07, -43.7232) -> (17.44, -40.9)
  line L328 (23.96, -40.9) -> (24.96, -40.9)
  line L329 (24.96, -40.9) -> (26.59, -38.0768)
  line L330 (26.59, -38.0768) -> (29.85, -38.0768)
  line L331 (29.85, -38.0768) -> (31.48, -40.9)
  line L332 (31.48, -40.9) -> (29.85, -43.7232)
  line L333 (29.85, -43.7232) -> (26.59, -43.7232)
  line L334 (26.59, -43.7232) -> (24.96, -40.9)
  line L335 (31.48, -40.9) -> (32.48, -40.9)
  line L336 (2.4, -40.9) -> (0, -40.9)
  line L337 (34.11, -43.7232) -> (32.48, -40.9)
  line L338 (32.48, -40.9) -> (34.11, -38.0768)
  line L339 (37.37, -43.7232) -> (34.11, -43.7232)
  line L340 (34.11, -38.0768) -> (37.37, -38.0768)
  line L341 (37.37, -38.0768) -> (39, -40.9)
  line L342 (39, -40.9) -> (37.37, -43.7232)
  line L343 (39, -40.9) -> (40, -40.9)
  line L344 (4.03, -38.0768) -> (37.37, -38.0768)
  line L345 (4.03, -43.7232) -> (37.37, -43.7232)
  line L346 (2.4, -51.3465) -> (4.03, -48.5232)
  line L347 (4.03, -48.5232) -> (7.29, -48.5232)
  line L348 (7.29, -48.5232) -> (8.92, -51.3465)
  line L349 (8.92, -51.3465) -> (7.29, -54.1697)
  line L350 (7.29, -54.1697) -> (4.03, -54.1697)
  line L351 (4.03, -54.1697) -> (2.4, -51.3465)
  line L352 (8.92, -51.3465) -> (9.92, -51.3465)
  line L353 (9.92, -51.3465) -> (11.55, -48.5232)
  line L354 (11.55, -48.5232) -> (14.81, -48.5232)
  line L355 (14.81, -48.5232) -> (16.44, -51.3465)
  line L356 (16.44, -51.3465) -> (14.81, -54.1697)
  line L357 (14.81, -54.1697) -> (11.55, -54.1697)
  line L358 (11.55, -54.1697) -> (9.92, -51.3465)
  line L359 (16.44, -51.3465) -> (17.44, -51.3465)
  line L360 (17.44, -51.3465) -> (19.07, -48.5232)
  line L361 (19.07, -48.5232) -> (22.33, -48.5232)
  line L362 (22.33, -48.5232) -> (23.96, -51.3465)
  line L363 (23.96, -51.3465) -> (22.33, -54.1697)
  line L364 (22.33, -54.1697) -> (19.07, -54.1697)
  line L365 (19.07, -54.1697) -> (17.44, -51.3465)
  line L366 (23.96, -51.3465) -> (24.96, -51.3465)
  line L367 (24.96, -51.3465) -> (26.59, -48.5232)
  line L368 (26.59, -48.5232) -> (29.85, -48.5232)
  line L369 (29.85, -48.5232) -> (31.48, -51.3465)
  line L370 (31.48, -51.3465) -> (29.85, -54.1697)
  line L371 (29.85, -54.1697) -> (26.59, -54.1697)
  line L372 (26.59, -54.1697) -> (24.96, -51.3465)
  line L373 (31.48, -51.3465) -> (32.48, -51.3465)
  line L374 (2.4, -51.3465) -> (0, -51.3465)
  line L375 (34.11, -54.1697) -> (32.48, -51.3465)
  line L376 (32.48, -51.3465) -> (34.11, -48.5232)
  line L377 (37.37, -54.1697) -> (34.11, -54.1697)
  line L378 (34.11, -48.5232) -> (37.37, -48.5232)
  line L379 (37.37, -48.5232) -> (39, -51.3465)
  line L380 (39, -51.3465) -> (37.37, -54.1697)
  line L381 (39, -51.3465) -> (40, -51.3465)
  line L382 (4.03, -48.5232) -> (37.37, -48.5232)
  line L383 (4.03, -54.1697) -> (37.37, -54.1697)
  line L384 (2.4, -61.793) -> (4.03, -58.9697)
  line L385 (4.03, -58.9697) -> (7.29, -58.9697)
  line L386 (7.29, -58.9697) -> (8.92, -61.793)
  line L387 (8.92, -61.793) -> (7.29, -64.6162)
  line L388 (7.29, -64.6162) -> (4.03, -64.6162)
  line L389 (4.03, -64.6162) -> (2.4, -61.793)
  line L390 (8.92, -61.793) -> (9.92, -61.793)
  line L391 (9.92, -61.793) -> (11.55, -58.9697)
  line L392 (11.55, -58.9697) -> (14.81, -58.9697)
  line L393 (14.81, -58.9697) -> (16.44, -61.793)
  line L394 (16.44, -61.793) -> (14.81, -64.6162)
  line L395 (14.81, -64.6162) -> (11.55, -64.6162)
  line L396 (11.55, -64.6162) -> (9.92, -61.793)
  line L397 (16.44, -61.793) -> (17.44, -61.793)
  line L398 (17.44, -61.793) -> (19.07, -58.9697)
  line L399 (19.07, -58.9697) -> (22.33, -58.9697)
  line L400 (22.33, -58.9697) -> (23.96, -61.793)
  line L401 (23.96, -61.793) -> (22.33, -64.6162)
  line L402 (22.33, -64.6162) -> (19.07, -64.6162)
  line L403 (19.07, -64.6162) -> (17.44, -61.793)
  line L404 (23.96, -61.793) -> (24.96, -61.793)
  line L405 (24.96, -61.793) -> (26.59, -58.9697)
  line L406 (26.59, -58.9697) -> (29.85, -58.9697)
  line L407 (29.85, -58.9697) -> (31.48, -61.793)
  line L408 (31.48, -61.793) -> (29.85, -64.6162)
  line L409 (29.85, -64.6162) -> (26.59, -64.6162)
  line L410 (26.59, -64.6162) -> (24.96, -61.793)
  line L411 (31.48, -61.793) -> (32.48, -61.793)
  line L412 (2.4, -61.793) -> (0, -61.793)
  line L413 (34.11, -64.6162) -> (32.48, -61.793)
  line L414 (32.48, -61.793) -> (34.11, -58.9697)
  line L415 (37.37, -64.6162) -> (34.11, -64.6162)
  line L416 (34.11, -58.9697) -> (37.37, -58.9697)
  line L417 (37.37, -58.9697) -> (39, -61.793)
  line L418 (39, -61.793) -> (37.37, -64.6162)
  line L419 (39, -61.793) -> (40, -61.793)
  line L420 (4.03, -58.9697) -> (37.37, -58.9697)
  line L421 (4.03, -64.6162) -> (37.37, -64.6162)
  line L422 (2.4, -72.2395) -> (4.03, -69.4162)
  line L423 (4.03, -69.4162) -> (7.29, -69.4162)
  line L424 (7.29, -69.4162) -> (8.92, -72.2395)
  line L425 (8.92, -72.2395) -> (7.29, -75.0627)
  line L426 (7.29, -75.0627) -> (4.03, -75.0627)
  line L427 (4.03, -75.0627) -> (2.4, -72.2395)
  line L428 (8.92, -72.2395) -> (9.92, -72.2395)
  line L429 (9.92, -72.2395) -> (11.55, -69.4162)
  line L430 (11.55, -69.4162) -> (14.81, -69.4162)
  line L431 (14.81, -69.4162) -> (16.44, -72.2395)
  line L432 (16.44, -72.2395) -> (14.81, -75.0627)
  line L433 (14.81, -75.0627) -> (11.55, -75.0627)
  line L434 (11.55, -75.0627) -> (9.92, -72.2395)
  line L435 (16.44, -72.2395) -> (17.44, -72.2395)
  line L436 (17.44, -72.2395) -> (19.07, -69.4162)
  line L437 (19.07, -69.4162) -> (22.33, -69.4162)
  line L438 (22.33, -69.4162) -> (23.96, -72.2395)
  line L439 (23.96, -72.2395) -> (22.33, -75.0627)
  line L440 (22.33, -75.0627) -> (19.07, -75.0627)
  line L441 (19.07, -75.0627) -> (17.44, -72.2395)
  line L442 (23.96, -72.2395) -> (24.96, -72.2395)
  line L443 (24.96, -72.2395) -> (26.59, -69.4162)
  line L444 (26.59, -69.4162) -> (29.85, -69.4162)
  line L445 (29.85, -69.4162) -> (31.48, -72.2395)
  line L446 (31.48, -72.2395) -> (29.85, -75.0627)
  line L447 (29.85, -75.0627) -> (26.59, -75.0627)
  line L448 (26.59, -75.0627) -> (24.96, -72.2395)
  line L449 (31.48, -72.2395) -> (32.48, -72.2395)
  line L450 (2.4, -72.2395) -> (0, -72.2395)
  line L451 (34.11, -75.0627) -> (32.48, -72.2395)
  line L452 (32.48, -72.2395) -> (34.11, -69.4162)
  line L453 (37.37, -75.0627) -> (34.11, -75.0627)
  line L454 (34.11, -69.4162) -> (37.37, -69.4162)
  line L455 (37.37, -69.4162) -> (39, -72.2395)
  line L456 (39, -72.2395) -> (37.37, -75.0627)
  line L457 (39, -72.2395) -> (40, -72.2395)
  line L458 (4.03, -69.4162) -> (37.37, -69.4162)
  line L459 (4.03, -75.0627) -> (37.37, -75.0627)
  line L460 (4.03, -79.8627) -> (14.81, -79.8627)
  line L461 (14.81, -85.5092) -> (4.03, -85.5092)
  point P0 (37.4, -4.8)
  point P1 (5.66, -9.5605)
  point P2 (5.66, -20.007)
  point P3 (5.66, -30.4535)
  point P4 (5.66, -40.9)
  point P5 (5.66, -51.3465)
  point P6 (5.66, -61.793)
  point P7 (5.66, -72.2395)
  point P8 (5.66, -82.6859)
  point P9 (9.92, -30.2362)
  point P10 (13.18, -9.5605)
  point P11 (13.18, -20.007)
  point P12 (13.18, -30.4535)
  point P13 (13.18, -40.9)
  point P14 (13.18, -51.3465)
  point P15 (13.18, -61.793)
  point P16 (13.18, -72.2395)
  point P17 (13.18, -82.6859)
  point P18 (17.44, -30.2362)
  point P19 (20.7, -9.5605)
  point P20 (20.7, -20.007)
  point P21 (20.7, -30.4535)
  point P22 (20.7, -40.9)
  point P23 (20.7, -51.3465)
  point P24 (20.7, -61.793)
  point P25 (20.7, -72.2395)
  point P26 (24.96, -30.2362)
  point P27 (28.22, -9.5605)
  point P28 (28.22, -20.007)
  point P29 (28.22, -30.4535)
  point P30 (28.22, -40.9)
  point P31 (28.22, -51.3465)
  point P32 (28.22, -61.793)
  point P33 (28.22, -72.2395)
  point P34 (35.74, -30.4535)
  point P35 (35.74, -40.9)
  point P36 (32.48, -30.2362)
  point P37 (35.74, -51.3465)
  point P38 (35.74, -61.793)
  point P39 (35.74, -72.2395)
  point P40 (35.74, -9.5605)
  point P41 (35.74, -20.007)
  point P42 (5.66, -20.007)
  point P43 (13.18, -20.007)
  point P44 (20.7, -20.007)
  point P45 (28.22, -20.007)
  point P46 (35.74, -20.007)
  point P47 (5.66, -30.4535)
  point P48 (13.18, -30.4535)
  point P49 (20.7, -30.4535)
  point P50 (28.22, -30.4535)
  point P51 (35.74, -30.4535)
  point P52 (5.66, -40.9)
  point P53 (13.18, -40.9)
  point P54 (20.7, -40.9)
  point P55 (28.22, -40.9)
  point P56 (35.74, -40.9)
  point P57 (5.66, -51.3465)
  point P58 (13.18, -51.3465)
  point P59 (20.7, -51.3465)
  point P60 (28.22, -51.3465)
  point P61 (35.74, -51.3465)
  point P62 (5.66, -61.793)
  point P63 (13.18, -61.793)
  point P64 (20.7, -61.793)
  point P65 (28.22, -61.793)
  point P66 (35.74, -61.793)
  point P67 (5.66, -72.2395)
  point P68 (13.18, -72.2395)
  point P69 (20.7, -72.2395)
  point P70 (28.22, -72.2395)
  point P71 (35.74, -72.2395)
  point P72 (11.55, -69.4162)
  point P73 (14.81, -69.4162)
  point P74 (14.81, -75.0627)
  point P75 (26.59, -75.0627)
  point P76 (34.11, -58.9697)
  point P77 (29.85, -58.9697)
  point P78 (29.85, -64.6162)
  point P79 (34.11, -64.6162)
  point P80 (26.59, -64.6162)
  point P81 (26.59, -58.9697)
  point P82 (29.85, -54.1697)
  point P83 (34.11, -54.1697)
  point P84 (14.81, -54.1697)
  point P85 (11.55, -54.1697)
  point P86 (11.55, -48.5232)
  point P87 (22.33, -54.1697)
  point P88 (29.85, -12.3838)
  point P89 (34.11, -6.7373)
  point P90 (29.85, -6.7373)
  point P91 (11.55, -6.7373)
  point P92 (7.29, -6.7373)
  point P93 (7.29, -12.3838)
  point P94 (19.07, -6.7373)
  point P95 (14.81, -6.7373)
  point P96 (14.81, -12.3838)
  point P97 (26.59, -6.7373)
  point P98 (22.33, -6.7373)
  point P99 (22.33, -12.3838)
  point P100 (26.59, -12.3838)
  point P101 (14.81, -17.1838)
  point P102 (26.59, -22.8303)
  point P103 (22.33, -17.1838)
  point P104 (29.85, -22.8303)
  point P105 (34.11, -22.8303)
  point P106 (34.11, -17.1838)
  point P107 (29.85, -17.1838)
  point P108 (11.55, -22.8303)
  point P109 (11.55, -17.1838)
  point P110 (14.81, -43.7232)
  point P111 (22.33, -43.7232)
  point P112 (26.59, -38.0768)
  point P113 (29.85, -43.7232)
  point P114 (34.11, -38.0768)
  point P115 (29.85, -38.0768)
  point P116 (11.55, -43.7232)
  point P117 (11.55, -38.0768)
  point P118 (7.29, -38.0768)
  point P119 (26.59, -33.2768)
  point P120 (26.59, -27.6303)
  point P121 (19.07, -27.6303)
  point P122 (14.81, -27.6303)
  point P123 (34.11, -27.6303)
  point P124 (29.85, -27.6303)
  point P125 (29.85, -33.2768)
  constraints: 924 end point, 9 horizontal, 1 parallel, 871 other
extrude "Extrusão16" cut sketch "Esboço24" against normal blind 10